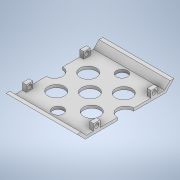
# Autodesk Inventor part: Bed
Saved by Autodesk Inventor 2021 (Build 250183000, 183)
## iProperties
Created: 2021-08-13
Part Number: Bed
Material: Generic
Document SubType Name: Modeling
Designer: rbnsmathew
Density: 1 g/cm^3
Appearance: Default
Mass: 14.9909 g
Surface Area: 131.725 cm^2
Volume: 14.9909 cm^3
Author: rbnsmathew
Autodesk Inventor part; units mm, degrees
ref_plane "YZ Plane" through (0, 0, 0) normal (1, 0, 0) x (0, 1, 0)
ref_plane "XZ Plane" through (0, 0, 0) normal (0, 1, 0) x (-1, 0, 0)
ref_plane "XY Plane" through (0, 0, 0) normal (0, 0, 1) x (1, 0, 0)
sketch "Sketch1" plane through (0, 0, 0) normal (1, 0, 0) x (0, 1, 0)
  line L0 (21.7077, 51.1019) -> (7.4012, 36.7954)
  line L1 (7.4012, 36.7954) -> (7.4012, 0)
  line L2 (21.7077, 51.1019) -> (21.7077, 0)
  line L3 (7.4012, -36.7954) -> (7.4012, 0)
  line L4 (21.7077, -51.1019) -> (21.7077, 0)
  line L5 (21.7077, -51.1019) -> (7.4012, -36.7954)
  line L6 (21.7077, -51.1019) -> (21.7077, 51.1019)
  line L7 (17.1717, -14.2524) -> (13.4217, -14.2524)
  line L8 (13.4217, -14.2524) -> (11.5467, -17.5)
  line L9 (19.0467, -17.5) -> (17.1717, -14.2524)
  circle A0 centre (15.2967, -17.5) radius 3.75
  line L10 (17.1717, -20.7476) -> (19.0467, -17.5)
  line L11 (11.5467, -17.5) -> (13.4217, -20.7476)
  line L12 (13.4217, -20.7476) -> (17.1717, -20.7476)
  line L13 (17.1717, -31.7524) -> (13.4217, -31.7524)
  line L14 (19.0467, -35) -> (17.1717, -31.7524)
  line L15 (13.4217, -31.7524) -> (11.5467, -35)
  line L16 (13.4217, -38.2476) -> (17.1717, -38.2476)
  line L17 (17.1717, -38.2476) -> (19.0467, -35)
  line L18 (11.5467, -35) -> (13.4217, -38.2476)
  circle A1 centre (15.2967, -35) radius 3.75
  circle A2 centre (15.2967, 0) radius 3.75
  line L19 (13.4217, -3.2476) -> (17.1717, -3.2476)
  line L20 (17.1717, -3.2476) -> (19.0467, 0)
  line L21 (11.5467, 0) -> (13.4217, -3.2476)
  line L22 (13.4217, 3.2476) -> (11.5467, 0)
  line L23 (17.1717, 3.2476) -> (13.4217, 3.2476)
  line L24 (19.0467, 0) -> (17.1717, 3.2476)
  line L25 (13.4217, 14.2524) -> (17.1717, 14.2524)
  line L26 (11.5467, 17.5) -> (13.4217, 14.2524)
  line L27 (17.1717, 14.2524) -> (19.0467, 17.5)
  circle A3 centre (15.2967, 17.5) radius 3.75
  line L28 (19.0467, 17.5) -> (17.1717, 20.7476)
  line L29 (17.1717, 20.7476) -> (13.4217, 20.7476)
  line L30 (13.4217, 20.7476) -> (11.5467, 17.5)
  circle A4 centre (15.2967, 35) radius 3.75
  line L31 (13.4217, 31.7524) -> (17.1717, 31.7524)
  line L32 (11.5467, 35) -> (13.4217, 31.7524)
  line L33 (17.1717, 31.7524) -> (19.0467, 35)
  line L34 (19.0467, 35) -> (17.1717, 38.2476)
  line L35 (13.4217, 38.2476) -> (11.5467, 35)
  line L36 (17.1717, 38.2476) -> (13.4217, 38.2476)
  line L37 (21.7077, 47.5664) -> (7.4012, 33.2599)
  line L38 (9.9012, 39.2954) -> (9.9012, -39.2954)
  line L39 (7.4012, -33.2599) -> (21.7077, -47.5664)
  line L40 (15.2967, 35) -> (9.9012, 35)
  line L41 (9.9012, 26.25) -> (16.1703, 26.25)
  circle A5 centre (12.9012, 26.25) radius 2
  line L42 (9.9012, 23.25) -> (15.9012, 23.25)
  line L43 (15.9012, 23.25) -> (15.9012, 29.25)
  line L44 (15.9012, 29.25) -> (9.9012, 29.25)
  line L45 (9.9012, 29.25) -> (9.9012, 23.25)
  line L46 (9.9012, 23.25) -> (15.9012, 29.25) construction
  line L47 (15.9012, 23.25) -> (9.9012, 29.25) construction
  line L48 (9.9012, -26.25) -> (17.1717, -26.25)
  circle A6 centre (12.9012, -26.25) radius 2
  line L49 (15.9012, -29.25) -> (9.9012, -29.25)
  line L50 (9.9012, -29.25) -> (9.9012, -23.25)
  line L51 (9.9012, -23.25) -> (15.9012, -23.25)
  line L52 (15.9012, -23.25) -> (15.9012, -29.25)
  line L53 (15.9012, -29.25) -> (9.9012, -23.25) construction
  line L54 (9.9012, -29.25) -> (15.9012, -23.25) construction
  line L55 (15.9012, 53.3729) -> (15.9012, -51.1019)
  line L56 (9.9012, 26.25) -> (7.4012, 26.25)
  line L57 (14.9012, -60.8562) -> (14.9012, 66.1701)
  point P0 (9.9012, 35.7599)
  point P1 (9.9012, -35.7599)
  point P2 (14.9012, 40.7599)
  point P3 (14.9012, 44.2954)
  point P4 (14.9012, -44.2954)
  point P5 (14.9012, -40.7599)
  dimension "d33" = 2.5
  dimension "d34" = 2.5
  dimension "d35" = 2.5
  dimension "d36" = 8.75
  dimension "d37" = 4
  dimension "d38" = 3
  dimension "d39" = 6
  dimension "d40" = 8.75
  dimension "d41" = 4
  dimension "d42" = 3
  dimension "d43" = 6
  dimension "d48" = 8.5
  dimension "d49" = 7.5
  constraints: 116 end point, 14 horizontal, 13 point on line, 8 vertical, 7 parallel, 6 coincident, 5 horizontal alignment, 5 midpoint, 4 perpendicular, 2 centre point, 1 collinear, 75 other
  measures "d33" distance between parallel lines of L37 L0
  measures "d34" distance from line of L38 L1.end
  measures "d35" distance between parallel lines of L39 L5
  measures "d36" distance between parallel lines of L41 L40
  measures "d37" diameter of A5
  measures "d38" distance of L41.start A5.centre
  measures "d39" distance between parallel lines of L42 L44
  measures "d40" distance from line of L48 point (15.297, -35)
  measures "d41" diameter of A6
  measures "d42" distance of L48.start A6.centre
  measures "d43" distance between parallel lines of L51 L49
  measures "d48" distance between parallel lines of L55 L1
  measures "d49" distance between parallel lines of L57 L3
extrude "Extrusion1" add sketch "Sketch1" along normal blind 3.5 contours L38 L37 L1 L0 | L0 L57 L37 L38 | L38 L56 L1 L37 | L56 L38 L39 L3 L1 | L44 L57 A5 L41 L38 | L41 A5 L57 L42 L38 | L44 L43 L41 L57 | L39 L38 L5 L3 | L41 L43 L42 L57 | L39 L57 L5 L38 | L51 L57 A6 L48 L38 | L38 L48 A6 L57 L49 | L51 L52 L48 L57 | L57 L48 L52 L49
sketch "Sketch2" plane through (3.5, 0, 0) normal (1, 0, 0) x (0, 0, -1)
  line L0 (-44.2954, 14.9012) -> (-36.7954, 7.4012) projected
  line L1 (-36.7954, 7.4012) -> (36.7954, 7.4012) projected
  line L2 (36.7954, 7.4012) -> (44.2954, 14.9012) projected
  line L3 (40.7599, 14.9012) -> (35.7599, 9.9012) projected
  line L4 (35.7599, 9.9012) -> (29.25, 9.9012) projected
  line L5 (29.25, 9.9012) -> (29.25, 15.9012) projected
  line L6 (29.25, 15.9012) -> (23.25, 15.9012) projected
  line L7 (23.25, 15.9012) -> (23.25, 9.9012) projected
  line L8 (23.25, 9.9012) -> (-23.25, 9.9012) projected
  line L9 (-23.25, 9.9012) -> (-23.25, 15.9012) projected
  line L10 (-23.25, 15.9012) -> (-29.25, 15.9012) projected
  line L11 (-29.25, 15.9012) -> (-29.25, 9.9012) projected
  line L12 (-29.25, 9.9012) -> (-35.7599, 9.9012) projected
  line L13 (-35.7599, 9.9012) -> (-40.7599, 14.9012) projected
  circle A0 centre (-26.25, 12.9012) radius 2 projected
  circle A1 centre (26.25, 12.9012) radius 2 projected
  line L14 (-29.25, 9.9012) -> (-23.25, 9.9012)
  line L15 (35.7599, 9.9012) -> (29.25, 9.9012) projected
  line L16 (23.25, 15.9012) -> (23.25, 9.9012) projected
  line L17 (29.25, 9.9012) -> (23.25, 9.9012)
  line L18 (-40.7599, 14.9012) -> (-44.2954, 14.9012) projected
  line L19 (44.2954, 14.9012) -> (40.7599, 14.9012) projected
  point P0 (0, 0)
  constraints: 4 end point, 2 horizontal
extrude "Extrusion2" add sketch "Sketch2" along normal blind 29 contours L18 L13 L12 L14 L8 L17 L4 L3 L19 L2 L1 L0
mirror "Mirror1" about plane through (32.5, 11.1512, 0) normal (1, 0, 0)
sketch "Sketch4" plane through (0, 9.9012, 23.25) normal (0, 1, 0) x (1, 0, 0)
  line L0 (0, 59.0099) -> (0, 52.5) projected
  line L1 (0, 52.5) -> (3.5, 52.5) projected
  line L2 (3.5, 46.5) -> (3.5, 52.5) projected
  line L3 (0, 46.5) -> (3.5, 46.5) projected
  line L4 (0, 46.5) -> (0, 0) projected
  line L5 (0, 0) -> (3.5, 0) projected
  line L6 (3.5, -6) -> (3.5, 0) projected
  line L7 (0, -6) -> (3.5, -6) projected
  line L8 (0, -6) -> (0, -12.5099) projected
  line L9 (0, -12.5099) -> (65, -12.5099) projected
  line L10 (65, -6) -> (65, -12.5099) projected
  line L11 (65, -6) -> (61.5, -6) projected
  line L12 (61.5, -6) -> (61.5, 0) projected
  line L13 (65, 0) -> (61.5, 0) projected
  line L14 (65, 46.5) -> (65, 0) projected
  line L15 (65, 46.5) -> (61.5, 46.5) projected
  line L16 (61.5, 46.5) -> (61.5, 52.5) projected
  line L17 (65, 52.5) -> (61.5, 52.5) projected
  line L18 (65, 59.0099) -> (65, 52.5) projected
  line L19 (0, 59.0099) -> (65, 59.0099) projected
  line L20 (0, 52.5) -> (65, 52.5)
  line L21 (65, -13.5454) -> (65, 60.0454) projected
  line L22 (0, -6) -> (65, -6)
  line L23 (0, 52.5) -> (65, -6)
  line L24 (0, -6) -> (3.5, -6) projected
  line L25 (0, -6) -> (65, 52.5)
  line L26 (32.5, 52.5) -> (32.5, -6)
  line L27 (65, 46.5) -> (65, 0) projected
  line L28 (65, 23.25) -> (0, 23.25)
  line L29 (65, 23.25) -> (32.5, 52.5)
  line L30 (0, 23.25) -> (32.5, 52.5)
  line L31 (0, 23.25) -> (32.5, -6)
  line L32 (32.5, -6) -> (65, 23.25)
  circle A0 centre (16.25, 37.875) radius 7.5
  circle A1 centre (32.5, 23.25) radius 7.5
  circle A2 centre (48.75, 37.875) radius 7.5
  circle A3 centre (16.25, 8.625) radius 7.5
  circle A4 centre (48.75, 8.625) radius 7.5
  line L33 (16.25, 59.0099) -> (16.25, -12.5099)
  line L34 (0, -12.5099) -> (65, -12.5099) projected
  line L35 (48.75, -12.5099) -> (48.75, 59.0099)
  line L36 (0, 59.0099) -> (65, 59.0099) projected
  line L37 (32.5, 59.0099) -> (32.5, -12.5099)
  circle A5 centre (32.5, 52.5) radius 5
  circle A6 centre (32.5, -6) radius 5
  arc A7 (0, 15.75) -> (0, 30.75) centre (0, 23.25) ccw
  arc A8 (65, 30.75) -> (65, 15.75) centre (65, 23.25) ccw
  dimension "d62" = 15
  dimension "d63" = 15
  dimension "d64" = 15
  dimension "d65" = 15
  dimension "d66" = 15
  dimension "d69" = 10
  dimension "d70" = 10
  dimension "d71" = 15
  dimension "d72" = 15
  constraints: 26 end point, 11 midpoint, 9 centre point, 8 point on line, 5 parallel, 4 coincident, 4 point on circle, 3 perpendicular
  measures "d62" diameter of A0
  measures "d63" diameter of A1
  measures "d64" diameter of A3
  measures "d65" diameter of A4
  measures "d66" diameter of A2
  measures "d69" diameter of A6
  measures "d70" diameter of A5
  measures "d71" diameter of A7
  measures "d72" diameter of A8
extrude "Extrusion3" cut sketch "Sketch4" against normal blind 10 contours A0 L33 L23 | L23 L30 A0 | A5 L20 L37 | L37 L20 A5 | L20 L30 A5 | A0 L30 L33 | L30 A0 L23 | L33 A0 L30 | L23 A0 L33 | L29 A5 L26 | L20 A5 L29 | L26 A5 L30 | A7 L30 L4 | A7 L28 L30 | L35 L29 A2 | A2 L25 L35 | L31 A7 L4 | L28 A7 L31 | A1 L26 L23 | L23 L28 A1 | A2 L29 L25 | L29 L25 A2 | L35 A2 L25 | L29 A2 L35 | A1 L25 L26 | L28 A1 L23 | L26 A1 L25 | L23 A1 L26 | L25 A1 L28 | L25 A1 L28 | L33 L31 A3 | A3 L25 L33 | L14 L29 A8 | L31 L25 A3 | A3 L31 L25 | L33 A3 L25 | L31 A3 L33 | L32 A8 L28 | L28 A8 L29 | L14 A8 L32 | A4 L35 L23 | L23 L32 A4 | A6 L32 L26 | L26 L31 A6 | A4 L32 L35 | L32 A4 L23 | L35 A4 L32 | L23 A4 L35 | L32 A6 L22 | L37 A6 L22 | L22 A6 L31 | L22 A6 L37
body "Solid1"
